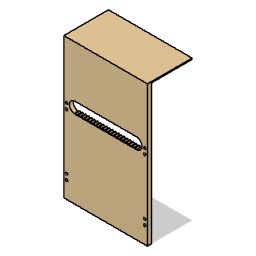
extension (left and right) v16 (Autodesk Fusion 360 design; units mm, degrees)
Autodesk Fusion 360 part; units mm, degrees
sketch "Sketch1" plane through (0, 0, 0) normal (0, 1, 0) x (1, 0, 0)
  line L0 (0, 0) -> (0, -7)
  line L1 (0, -7) -> (-150, -7)
  line L2 (-150, -7) -> (-150, 0)
  line L3 (-150, 0) -> (0, 0)
  dimension "d1" = 7
  dimension "d2" = 150
  constraint coincident L0.start L3.end
  constraint vertical L0
  constraint perpendicular L0 L1
  constraint perpendicular L1 L2
  constraint perpendicular L0 L3
  measures "d1" distance of L0.start L0.end
  measures "d2" distance of L0.end L1.end
extrude "Extrude1" add sketch "Sketch1" against normal blind 252 makes body 1
sketch "Sketch2" plane through (0, 0, 0) normal (1, 0, 0) x (0, 0, -1)
  line L0 (0, 0) -> (73, 0)
  line L1 (73, 0) -> (73, -2)
  line L2 (73, -2) -> (0, -2)
  line L3 (0, -2) -> (0, 0)
  dimension "d5" = 73
  dimension "d6" = 2
  constraint horizontal L0
  constraint vertical L1
  constraint horizontal L2
  constraint vertical L3
  constraint coincident L0.start L3.end
  measures "d5" distance of L0.start L0.end
  measures "d6" distance of L2.end L0.start
extrude "Extrude2" add sketch "Sketch2" against normal blind 150 bodies 1
sketch "Sketch3" plane through (0, 0, 0) normal (0, 0, 1) x (1, 0, 0)
  circle A0 centre (-5, -112) radius 2.5
  circle A1 centre (-5, -102) radius 2.5
  line L0 (0, 0) -> (-150, 0)
  line L1 (0, 0) -> (0, -252)
  circle A2 centre (-145, -102) radius 2.5
  circle A3 centre (-145, -112) radius 2.5
  line L2 (-150, 0) -> (-150, -252)
  dimension "d9" = 102
  dimension "d10" = 10
  dimension "d11" = 5
  dimension "d12" = 5
  dimension "d71" = 5
  dimension "d72" = 5
  dimension "d73" = 5
  dimension "d74" = 10
  dimension "d75" = 5
  constraint horizontal A1.centre A2.centre
  constraint horizontal A0.centre A3.centre
  constraint vertical A2.centre A3.centre
  measures "d9" distance of A1.centre L0
  measures "d10" distance of A0.centre A1.centre
  measures "d11" diameter of A0
  measures "d12" diameter of A1
  measures "d16" radius of L0.end
  measures "d71" distance of A1.centre L1
  measures "d72" diameter of A2
  measures "d73" diameter of A3
  measures "d74" distance of A2.centre A3.centre
  measures "d75" distance of A2.centre L2
sketch "Sketch4" plane through (0, 0, 7) normal (0, 0, 1) x (1, 0, 0)
  line L0 (0, 0) -> (-150, 0)
  line L1 (-150, 0) -> (-150, -252)
  line L2 (-150, -252) -> (0, -252)
  line L3 (0, -252) -> (0, 0)
  line L4 (-130, -92) -> (-20, -92)
  line L5 (-130, -112) -> (-20, -112)
  arc A0 (-130, -92) -> (-130, -112) centre (-130, -102) ccw
  arc A1 (-20, -112) -> (-20, -92) centre (-20, -102) ccw
  point P0 (-5, -102)
  point P1 (-5, -112)
  dimension "d13" = 102
  dimension "d14" = 20
  dimension "d15" = 10
  dimension "d16" = 10
  dimension "d17" = 110
  dimension "d18" = 20
  dimension "d59" = 150
  constraint perpendicular L1 L4
  constraint perpendicular L1 L5
  constraint tangent L5 A0
  constraint tangent L4 A0
  constraint tangent L5 A1
  constraint tangent L4 A1
  measures "d13" vertical distance of L0.start A0.centre
  measures "d14" distance of L4 L5
  measures "d15" radius of A0
  measures "d16" radius of A1
  measures "d17" distance of L4.start L4.end
  measures "d18" horizontal distance of L0.start L4.end
  measures "d59" distance of L0.start L0.end
extrude "Extrude6" cut sketch "Sketch4" against normal blind 100 contours L4 L5 A0 A1 bodies 1
sketch "草图6" plane through (0, 0, 7) normal (0, 0, 1) x (1, 0, 0)
  line L0 (-20, -112) -> (-130, -112)
  arc A0 (-130, -92) -> (-130, -112) centre (-130, -102) ccw
  line L1 (-130, -92) -> (-20, -92)
  arc A1 (-20, -112) -> (-20, -92) centre (-20, -102) ccw
  line L2 (0, 0) -> (-150, 0)
  line L3 (-150, 0) -> (-150, -252)
  line L4 (-150, -252) -> (0, -252)
  line L5 (0, -252) -> (0, 0)
  line L6 (-130, -112) -> (-128.9739, -109.1809)
  line L7 (-130, -112) -> (-125.5798, -112) construction
  line L8 (-128.9739, -109.1809) -> (-127.9739, -109.1809)
  line L9 (-127.9739, -109.1809) -> (-126.9479, -112)
  line L10 (-127.9739, -109.1809) -> (-122.2899, -109.1809) construction
  line L11 (-130, -112) -> (-126.9479, -112)
  dimension "d43" = 3
  dimension "d44" = 70
  dimension "d45" = 1
  dimension "d46" = 70
  dimension "d47" = 3
  constraint horizontal L7
  constraint coincident L0.end A0.end
  constraint horizontal L8
  constraint horizontal L10
  measures "d43" distance of L0.end L6.end
  measures "d44" angle of L6 L7
  measures "d45" distance of L6.end L8.end
  measures "d46" angle of L9 L10
  measures "d47" distance of L8.end L9.end
extrude "拉伸7" add sketch "草图6" against normal blind 7 separate body contours L0 L6 L8 L9 L11 makes body 2
pattern_linear "R-阵列2" count 21 spacing 5.35 along (1, 0, 0) of "拉伸7" makes body 3 at (-122.6153, -112, 2.3333) makes body 4 at (-117.2653, -112, 2.3333) makes body 5 at (-111.9153, -112, 2.3333) makes body 6 at (-106.5653, -112, 2.3333) makes body 7 at (-95.8653, -112, 2.3333) makes body 8 at (-90.5153, -112, 2.3333) makes body 9 at (-85.1653, -112, 2.3333) makes body 10 at (-69.1153, -112, 2.3333) makes body 11 at (-101.2153, -112, 2.3333) makes body 12 at (-79.8153, -112, 2.3333) makes body 13 at (-74.4653, -112, 2.3333) makes body 14 at (-63.7653, -112, 2.3333) makes body 15 at (-58.4153, -112, 2.3333) makes body 16 at (-53.0653, -112, 2.3333) makes body 17 at (-47.7153, -112, 2.3333) makes body 18 at (-42.3653, -112, 2.3333) makes body 19 at (-37.0153, -112, 2.3333) makes body 20 at (-31.6653, -112, 2.3333) makes body 21 at (-26.3153, -112, 2.3333) makes body 22 at (-20.9653, -112, 2.3333)
sketch "草图7" plane through (0, 0, 7) normal (0, 0, 1) x (1, 0, 0)
  line L0 (-20, -112) -> (-130, -112)
  arc A0 (-130, -92) -> (-130, -112) centre (-130, -102) ccw
  line L1 (-130, -92) -> (-20, -92)
  arc A1 (-20, -112) -> (-20, -92) centre (-20, -102) ccw
  line L2 (0, 0) -> (-150, 0)
  line L3 (-150, 0) -> (-150, -252)
  line L4 (-150, -252) -> (0, -252)
  line L5 (0, -252) -> (0, 0)
  circle A2 centre (-5, -222) radius 2.5
  circle A3 centre (-5, -212) radius 2.5
  circle A4 centre (-145, -222) radius 2.5
  circle A5 centre (-145, -212) radius 2.5
  dimension "d60" = 5
  dimension "d61" = 5
  dimension "d62" = 5
  dimension "d63" = 5
  dimension "d64" = 10
  dimension "d65" = 30
  dimension "d66" = 5
  dimension "d67" = 5
  dimension "d68" = 5
  dimension "d69" = 5
  constraint horizontal A2.centre A4.centre
  constraint horizontal A3.centre A5.centre
  measures "d60" diameter of A2
  measures "d61" diameter of A3
  measures "d62" distance of L5 A2.centre
  measures "d63" distance of L5 A3.centre
  measures "d64" distance of A2.centre A3.centre
  measures "d65" distance of L4 A2.centre
  measures "d66" diameter of A4
  measures "d67" diameter of A5
  measures "d68" distance of L3 A4.centre
  measures "d69" distance of L3 A5.centre
extrude "拉伸8" cut sketch "草图7" against normal through all contours A2 | A3 | A4 | A5 bodies 1
extrude "拉伸9" cut sketch "Sketch3" along normal through all bodies 1
thread "螺纹1" "ISO Metric profile 5.0 M5x0.8 6H" major diameter 5.12 minor diameter 4.234 pitch 0.8 angle 60 resizes the face on face at (-144.2038, -209.6302, 2.3333) on bodies 1
thread "螺纹2" "ISO Metric profile 5.0 M5x0.8 6H" major diameter 5.12 minor diameter 4.234 pitch 0.8 angle 60 resizes the face on face at (-145.6771, -219.5934, 4.6667) on bodies 1
thread "螺纹3" "ISO Metric profile 5.0 M5x0.8 6H" major diameter 5.12 minor diameter 4.234 pitch 0.8 angle 60 resizes the face on face at (-2.5773, -212.6169, 4.6667) on bodies 1
thread "螺纹4" "ISO Metric profile 5.0 M5x0.8 6H" major diameter 5.12 minor diameter 4.234 pitch 0.8 angle 60 resizes the face on face at (-7.4227, -222.6169, 2.3333) on bodies 1
thread "螺纹5" "ISO Metric profile 5.0 M5x0.8 6H" major diameter 5.12 minor diameter 4.234 pitch 0.8 angle 60 resizes the face on face at (-144.2038, -99.6302, 2.3333) on face at (-144.2038, -109.6302, 2.3333) on face at (-7.3492, -111.1449, 4.6667) on face at (-7.3492, -101.1449, 4.6667) on bodies 1
